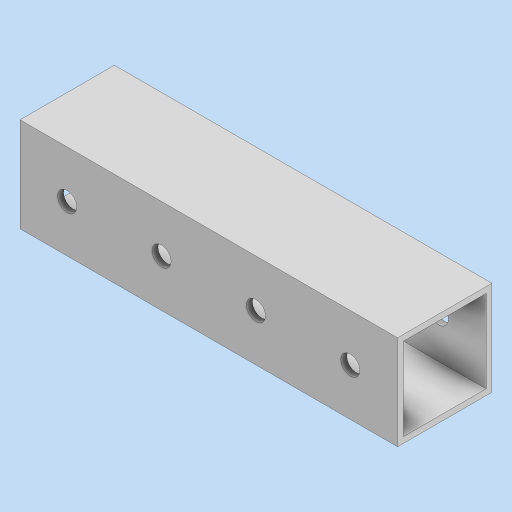
# Autodesk Inventor part: 1inTubeBase
Saved by Autodesk Inventor 2024 (Build 280153000, 153)
## iProperties
Created: 2024-01-10
Part Number: 1inTubeBase
Material: Generic
Document SubType Name: Modeling
Designer: megan
Density: 1 g/cm^3
Appearance: Default
Author: megan
Autodesk Inventor part; units mm, degrees
ref_plane "YZ Plane" through (0, 0, 0) normal (1, 0, 0) x (0, 1, 0)
ref_plane "XZ Plane" through (0, 0, 0) normal (0, 1, 0) x (-1, 0, 0)
ref_plane "XY Plane" through (0, 0, 0) normal (0, 0, 1) x (1, 0, 0)
sketch "Sketch1" plane through (0, 0, 0) normal (1, 0, 0) x (0, 1, 0)
  line L0 (0, 0) -> (25.4, 0)
  line L1 (25.4, 0) -> (25.4, -25.4)
  line L2 (25.4, -25.4) -> (0, -25.4)
  line L3 (0, -25.4) -> (0, 0)
  line L4 (23.8125, -23.8125) -> (23.8125, -1.5875)
  line L5 (23.8125, -1.5875) -> (1.5875, -1.5875)
  line L6 (1.5875, -1.5875) -> (1.5875, -23.8125)
  line L7 (1.5875, -23.8125) -> (23.8125, -23.8125)
  dimension "d0" = 25.4
  dimension "d1" = 25.4
  dimension "d2" = 1.5875
  constraints: 16 end point, 4 parallel, 2 perpendicular, 1 horizontal, 3 other
  measures "d0" distance of L1.end L2.end
  measures "d1" distance of L0.end L1.end
  measures "d2" distance between parallel lines of L1 L4
extrude "Extrusion1" add sketch "Sketch1" along normal mid plane 101.6
sketch "Sketch3" plane through (-50.8, 0, 0) normal (0, 0, 1) x (1, 0, 0)
  line L0 (0, 0) -> (101.6, 0) projected
  line L1 (101.6, 25.4) -> (101.6, 0) projected
  line L2 (0, 25.4) -> (101.6, 25.4) projected
  line L3 (0, 0) -> (0, 25.4) projected
  circle A0 centre (38.1, 12.7) radius 2.5781
  circle A1 centre (63.5, 12.7) radius 2.5781
  line L4 (50.8, 25.4) -> (50.8, 0) construction
  circle A2 centre (12.7, 12.7) radius 2.5781
  circle A3 centre (88.9, 12.7) radius 2.5781
  dimension "d14" = 5.1562
  dimension "d15" = 5.1562
  dimension "d16" = 12.7
  dimension "d17" = 25.4
  dimension "d20" = 12.7
  dimension "d21" = 25.4
  dimension "d22" = 25.4
  constraints: 4 centre point, 2 end point, 2 equal radius, 1 horizontal alignment, 1 midpoint, 1 vertical
  measures "d14" diameter of A0
  measures "d15" diameter of A1
  measures "d16" distance from line of L4 A0.centre
  measures "d17" distance of A1.centre A0.centre
  measures "d20" distance from line of L2 A0.centre
  measures "d21" distance of A2.centre A0.centre
  measures "d22" distance of A3.centre A1.centre
extrude "Extrusion3" cut sketch "Sketch3" against normal blind 25.4 contours A0 | A1 | A2 | A3
body "Solid1"
